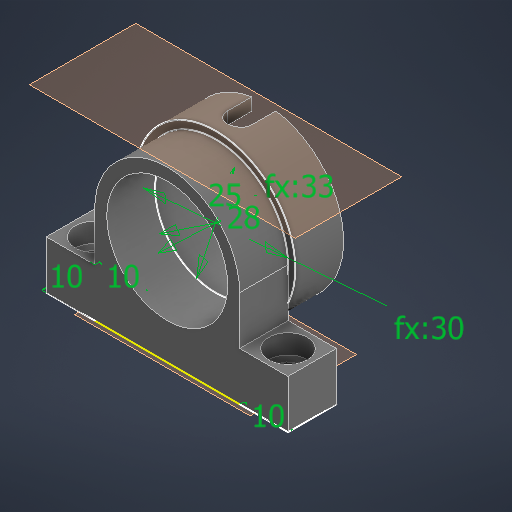
# Autodesk Inventor part: Adafruit_1528_4699_ND_House_01
Saved by Autodesk Inventor 2026.2 (Build 302298000, 298)
## iProperties
Created: 2026-02-02
Part Number: Adafruit_1528_4699_ND_House_01
Material: Generic
Document SubType Name: Modeling
Designer: vckot
Density: 1 g/cm^3
Appearance: Gray
Author: vckot
Autodesk Inventor part; units mm, degrees
ref_plane "YZ Plane" through (0, 0, 0) normal (1, 0, 0) x (0, 1, 0)
ref_plane "XY Plane" through (0, 0, 0) normal (0, 0, 1) x (1, 0, 0)
sketch "Sketch2" plane through (0, 0, 0) normal (0, 0, 1) x (1, 0, 0)
  circle A0 centre (0, 0) radius 14
  circle A1 centre (0, 0) radius 12.5
  circle A2 centre (0, 0) radius 16.5
  circle A3 centre (0, 0) radius 15
  dimension "d0" = 28
  dimension "d1" = 25
  dimension "d2" = 33
  dimension "d3" = 30
  constraints: 4 centre point, 4 coincident
  measures "d0" diameter of A0
  measures "d1" diameter of A1
  measures "d2" diameter of A2
  measures "d3" diameter of A3
extrude "Extrusion1" add sketch "Sketch2" against normal blind 10 contours A2 | A3
extrude "Extrusion2" add sketch "Sketch2" along normal blind 10 contours A0 | A3
ref_plane "Work Plane1" through (0, -20, 0) normal (0, 1, 0) x (-1, 0, 0)
sketch "Sketch3" plane through (0, -20, 0) normal (0, 1, 0) x (-1, 0, 0)
  line L0 (15, 10) -> (-15, 10) projected
  line L1 (-15, 0) -> (15, 0) projected
  line L2 (-15, 0) -> (-15, 10) projected
  line L3 (15, 0) -> (15, 10) projected
  line L4 (-15, 10) -> (-25, 10)
  line L5 (-25, 10) -> (-25, 0)
  line L6 (-25, 0) -> (-15, 0)
  line L7 (15, 10) -> (25, 10)
  line L8 (25, 10) -> (25, 0)
  line L9 (25, 0) -> (15, 0)
  line L10 (15, 0) -> (15, 10)
  point P0 (0, 0)
  dimension "d9" = 10
  dimension "d10" = 10
  dimension "d11" = 10
  constraints: 14 end point, 3 perpendicular, 2 horizontal, 2 parallel
  measures "d9" distance of L2.end L4.end
  measures "d10" distance of L8.end L9.end
  measures "d11" distance of L7.end L8.end
extrude "Extrusion3" add sketch "Sketch3" along normal through all contours L3 L1 L2 L0
extrude "Extrusion4" add sketch "Sketch3" along normal blind 10 contours L7 L8 L9 L3 | L2 L6 L5 L4
extrude "Extrusion5" cut sketch "Sketch2" along normal through all contours A1
sketch "Sketch4" plane through (0, -10, 0) normal (0, 1, 0) x (1, 0, 0)
  line L0 (25, -10) -> (25, 0) projected
  line L1 (15, -10) -> (25, -10) projected
  line L2 (-25, -10) -> (-15, -10) projected
  line L3 (-25, 0) -> (-25, -10) projected
  point P0 (0, 0)
  point P1 (20, -5)
  point P2 (-20, -5)
  dimension "d18" = 5
  dimension "d19" = 5
  dimension "d20" = 5
  dimension "d21" = 5
  measures "d18" distance from line of L0 point (20, -5)
  measures "d19" distance from line of L1 point (20, -5)
  measures "d20" distance from line of L2 point (-20, -5)
  measures "d21" distance from line of L3 point (-20, -5)
hole "Hole1" at (20, -10, 5) at (-20, -10, 5) direction (0, -1, 0) diameter 4.5 end through all counterbore diameter 8 counterbore depth 4 clearance for "Socket Head Cap Screw" size "M4" standard "Ansi Metric M Profile"
ref_plane "Work Plane2" through (0, 16.5, 0) normal (0, 1, 0) x (-1, 0, 0)
sketch "Sketch5" plane through (0, 16.5, 0) normal (0, 1, 0) x (-1, 0, 0)
  line L0 (-16.5, -10) -> (16.5, -10) projected
  line L1 (-2.5, -10) -> (2.5, -10)
  line L2 (2.5, -10) -> (2.5, -5)
  line L3 (2.5, -5) -> (-2.5, -5)
  line L4 (-2.5, -5) -> (-2.5, -10)
  arc A0 (2.5, -5) -> (-2.5, -5) centre (0, -5) ccw
  line L5 (16.5, 0) -> (-16.5, 0) projected
  point P0 (0, 0)
  point P1 (0, 0)
  point P2 (-15, 0)
  point P3 (15, 0)
  dimension "d29" = 2.5
  dimension "d30" = 5
  constraints: 8 end point, 2 midpoint, 2 parallel, 2 point on circle, 1 centre point, 1 horizontal, 1 perpendicular, 1 point on line, 1 vertical alignment
  measures "d29" radius of A0
  measures "d30" distance between parallel lines of L0 L3
extrude "Extrusion6" cut sketch "Sketch5" against normal blind 10
equation "\"d18\" = 0.5 * d9"
equation "\"d19\" = 0.5 * d9"
equation "\"d20\" = 0.5 * d11"
equation "\"d21\" = 0.5 * d11"
body "Solid1"
